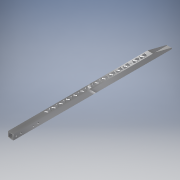
# Autodesk Inventor part: 15102898-16-P-0216
Saved by Autodesk Inventor 2017 (Build 210142000, 142)
## iProperties
Created: 2016-10-06
Part Number: 15102898-16-P-0216
Material: Aluminum 6061
Document SubType Name: Modeling
Designer: gus
Density: 2.7 g/cm^3
Appearance: Aluminum - Flat
Mass: 558.645 g
Surface Area: 1315.32 cm^2
Volume: 206.905 cm^3
Author: gus
Autodesk Inventor part; units mm, degrees
ref_plane "YZ Plane" through (0, 0, 0) normal (1, 0, 0) x (0, 1, 0)
ref_plane "XZ Plane" through (0, 0, 0) normal (0, 1, 0) x (-1, 0, 0)
ref_plane "XY Plane" through (0, 0, 0) normal (0, 0, 1) x (1, 0, 0)
sketch "Sketch1" plane through (0, 0, 0) normal (0, 0, 1) x (1, 0, 0)
  line L0 (0, 0) -> (-25.4, 0)
  line L1 (-25.4, 0) -> (-25.4, 25.4)
  line L2 (-25.4, 25.4) -> (0, 25.4)
  line L3 (0, 25.4) -> (0, 0)
  line L4 (-22.225, 22.225) -> (-22.225, 3.175)
  line L5 (-22.225, 3.175) -> (-3.175, 3.175)
  line L6 (-3.175, 3.175) -> (-3.175, 22.225)
  line L7 (-3.175, 22.225) -> (-22.225, 22.225)
  dimension "d0" = 25.4
  dimension "d1" = 25.4
  dimension "d2" = 3.175
  constraints: 16 end point, 4 parallel, 2 perpendicular, 1 horizontal, 3 other
  measures "d0" distance of L1.end L2.end
  measures "d1" distance of L0.end L1.end
  measures "d2" distance between parallel lines of L1 L4
extrude "Extrusion1" add sketch "Sketch1" along normal blind 736.6
sketch "Sketch2" plane through (-25.4, 25.4, 0) normal (0, 1, 0) x (1, 0, 0)
  circle A0 centre (12.7, -177.8) radius 3.175
  line L0 (0, 0) -> (0, -736.6) projected
  line L1 (0, 0) -> (25.4, 0) projected
  dimension "d5" = 6.35
  dimension "d6" = 12.7
  dimension "d7" = 177.8
  constraints: 1 centre point
  measures "d5" diameter of A0
  measures "d6" distance from line of L0 A0.centre
  measures "d7" distance from line of L1 A0.centre
extrude "Extrusion2" cut sketch "Sketch2" against normal blind 25.4
sketch "Sketch3" plane through (-25.4, 0, 0) normal (-1, 0, 0) x (0, 0, 1)
  circle A0 centre (723.9, 12.7) radius 3.175
  line L0 (0, 0) -> (736.6, 0) projected
  line L1 (736.6, 25.4) -> (736.6, 0) projected
  line L2 (736.6, 12.7) -> (584.2, 12.7) construction
  circle A1 centre (701.675, 12.7) radius 3.175
  circle A2 centre (644.525, 12.7) radius 3.175
  circle A3 centre (622.3, 12.7) radius 3.175
  dimension "d10" = 6.35
  dimension "d11" = 12.7
  dimension "d12" = 152.4
  dimension "d13" = 12.7
  dimension "d14" = 12.7
  dimension "d15" = 6.35
  dimension "d16" = 22.225
  dimension "d17" = 6.35
  dimension "d18" = 6.35
  dimension "d19" = 57.15
  dimension "d20" = 22.225
  constraints: 4 centre point, 3 point on line, 2 end point, 1 horizontal, 1 midpoint
  measures "d10" diameter of A0
  measures "d11" distance from line of L0 A0.centre
  measures "d12" distance of L2.start L2.end
  measures "d13" distance between parallel lines of L0 L2
  measures "d14" distance from line of L1 A0.centre
  measures "d15" diameter of A1
  measures "d16" distance of A0.centre A1.centre
  measures "d17" diameter of A2
  measures "d18" diameter of A3
  measures "d19" distance of A1.centre A2.centre
  measures "d20" distance of A3.centre A2.centre
extrude "Extrusion3" cut sketch "Sketch3" against normal blind 25.4
sketch "Sketch4" plane through (-25.4, 25.4, 0) normal (0, 1, 0) x (1, 0, 0)
  circle A0 centre (12.7, -723.9) radius 3.175
  circle A1 centre (12.7, -660.4) radius 3.175
  circle A2 centre (12.7, -596.9) radius 3.175
  line L0 (25.4, 0) -> (25.4, -736.6) projected
  line L1 (25.4, -736.6) -> (0, -736.6) projected
  circle A3 centre (12.7, -12.7) radius 3.175
  circle A4 centre (12.7, -92.075) radius 3.175
  line L2 (0, 0) -> (25.4, 0) projected
  line L3 (15.875, -581.4504) -> (6.2513, -575.8941)
  line L4 (6.2513, -570.3949) -> (15.875, -564.8386)
  line L5 (20.6375, -567.5882) -> (20.6375, -578.7007)
  line L6 (22.225, 0) -> (22.225, -736.6) projected
  line L7 (0, 0) -> (0, -736.6) projected
  line L8 (9.525, -564.8386) -> (19.1487, -559.2824)
  line L9 (19.1487, -553.7831) -> (9.525, -548.2268)
  line L10 (4.7625, -550.9765) -> (4.7625, -562.089)
  line L11 (22.225, 0) -> (3.175, 0) construction
  arc A5 (19.1487, -559.2824) -> (19.1487, -553.7831) centre (17.5612, -556.5327) ccw
  arc A6 (9.525, -548.2268) -> (4.7625, -550.9765) centre (7.9375, -550.9765) ccw
  arc A7 (4.7625, -562.089) -> (9.525, -564.8386) centre (7.9375, -562.089) ccw
  arc A8 (20.6375, -567.5882) -> (15.875, -564.8386) centre (17.4625, -567.5882) ccw
  arc A9 (15.875, -581.4504) -> (20.6375, -578.7007) centre (17.4625, -578.7007) ccw
  arc A10 (6.2513, -570.3949) -> (6.2513, -575.8941) centre (7.8388, -573.1445) ccw
  arc A11 (4.7625, -528.8404) -> (9.525, -531.59) centre (7.9375, -528.8404) ccw
  line L12 (4.7625, -517.7279) -> (4.7625, -528.8404)
  arc A12 (9.525, -514.9782) -> (4.7625, -517.7279) centre (7.9375, -517.7279) ccw
  arc A13 (6.2513, -537.1463) -> (6.2513, -542.6455) centre (7.8388, -539.8959) ccw
  arc A14 (20.6375, -534.3396) -> (15.875, -531.59) centre (17.4625, -534.3396) ccw
  line L13 (9.525, -531.59) -> (19.1487, -526.0338)
  line L14 (19.1487, -520.5345) -> (9.525, -514.9782)
  arc A15 (15.875, -548.2018) -> (20.6375, -545.4521) centre (17.4625, -545.4521) ccw
  line L15 (15.875, -548.2018) -> (6.2513, -542.6455)
  arc A16 (19.1487, -526.0338) -> (19.1487, -520.5345) centre (17.5612, -523.2841) ccw
  line L16 (20.6375, -534.3396) -> (20.6375, -545.4521)
  line L17 (6.2513, -537.1463) -> (15.875, -531.59)
  arc A17 (4.7625, -495.5918) -> (9.525, -498.3414) centre (7.9375, -495.5918) ccw
  line L18 (4.7625, -484.4793) -> (4.7625, -495.5918)
  arc A18 (9.525, -481.7296) -> (4.7625, -484.4793) centre (7.9375, -484.4793) ccw
  arc A19 (6.2513, -503.8977) -> (6.2513, -509.3969) centre (7.8388, -506.6473) ccw
  arc A20 (20.6375, -501.091) -> (15.875, -498.3414) centre (17.4625, -501.091) ccw
  line L19 (9.525, -498.3414) -> (19.1487, -492.7852)
  line L20 (19.1487, -487.2859) -> (9.525, -481.7296)
  arc A21 (15.875, -514.9532) -> (20.6375, -512.2035) centre (17.4625, -512.2035) ccw
  line L21 (15.875, -514.9532) -> (6.2513, -509.3969)
  arc A22 (19.1487, -492.7852) -> (19.1487, -487.2859) centre (17.5612, -490.0355) ccw
  line L22 (20.6375, -501.091) -> (20.6375, -512.2035)
  line L23 (6.2513, -503.8977) -> (15.875, -498.3414)
  arc A23 (4.7625, -462.3432) -> (9.525, -465.0928) centre (7.9375, -462.3432) ccw
  line L24 (4.7625, -451.2307) -> (4.7625, -462.3432)
  arc A24 (9.525, -448.481) -> (4.7625, -451.2307) centre (7.9375, -451.2307) ccw
  arc A25 (6.2513, -470.6491) -> (6.2513, -476.1483) centre (7.8388, -473.3987) ccw
  arc A26 (20.6375, -467.8424) -> (15.875, -465.0928) centre (17.4625, -467.8424) ccw
  line L25 (9.525, -465.0928) -> (19.1487, -459.5366)
  line L26 (19.1487, -454.0373) -> (9.525, -448.481)
  arc A27 (15.875, -481.7046) -> (20.6375, -478.9549) centre (17.4625, -478.9549) ccw
  line L27 (15.875, -481.7046) -> (6.2513, -476.1483)
  arc A28 (19.1487, -459.5366) -> (19.1487, -454.0373) centre (17.5612, -456.7869) ccw
  line L28 (20.6375, -467.8424) -> (20.6375, -478.9549)
  line L29 (6.2513, -470.6491) -> (15.875, -465.0928)
  arc A29 (4.7625, -429.0946) -> (9.525, -431.8442) centre (7.9375, -429.0946) ccw
  line L30 (4.7625, -417.9821) -> (4.7625, -429.0946)
  arc A30 (9.525, -415.2324) -> (4.7625, -417.9821) centre (7.9375, -417.9821) ccw
  arc A31 (6.2513, -437.4005) -> (6.2513, -442.8997) centre (7.8388, -440.1501) ccw
  arc A32 (20.6375, -434.5938) -> (15.875, -431.8442) centre (17.4625, -434.5938) ccw
  line L31 (9.525, -431.8442) -> (19.1487, -426.288)
  line L32 (19.1487, -420.7887) -> (9.525, -415.2324)
  arc A33 (15.875, -448.456) -> (20.6375, -445.7063) centre (17.4625, -445.7063) ccw
  line L33 (15.875, -448.456) -> (6.2513, -442.8997)
  arc A34 (19.1487, -426.288) -> (19.1487, -420.7887) centre (17.5612, -423.5383) ccw
  line L34 (20.6375, -434.5938) -> (20.6375, -445.7063)
  line L35 (6.2513, -437.4005) -> (15.875, -431.8442)
  arc A35 (4.7625, -395.846) -> (9.525, -398.5956) centre (7.9375, -395.846) ccw
  line L36 (4.7625, -384.7335) -> (4.7625, -395.846)
  arc A36 (9.525, -381.9838) -> (4.7625, -384.7335) centre (7.9375, -384.7335) ccw
  arc A37 (6.2513, -404.1519) -> (6.2513, -409.6511) centre (7.8388, -406.9015) ccw
  arc A38 (20.6375, -401.3452) -> (15.875, -398.5956) centre (17.4625, -401.3452) ccw
  line L37 (9.525, -398.5956) -> (19.1487, -393.0394)
  line L38 (19.1487, -387.5401) -> (9.525, -381.9838)
  arc A39 (15.875, -415.2074) -> (20.6375, -412.4577) centre (17.4625, -412.4577) ccw
  line L39 (15.875, -415.2074) -> (6.2513, -409.6511)
  arc A40 (19.1487, -393.0394) -> (19.1487, -387.5401) centre (17.5612, -390.2897) ccw
  line L40 (20.6375, -401.3452) -> (20.6375, -412.4577)
  line L41 (6.2513, -404.1519) -> (15.875, -398.5956)
  arc A41 (4.7625, -362.5974) -> (9.525, -365.347) centre (7.9375, -362.5974) ccw
  line L42 (4.7625, -351.4849) -> (4.7625, -362.5974)
  arc A42 (9.525, -348.7352) -> (4.7625, -351.4849) centre (7.9375, -351.4849) ccw
  arc A43 (6.2513, -370.9033) -> (6.2513, -376.4025) centre (7.8388, -373.6529) ccw
  arc A44 (20.6375, -368.0966) -> (15.875, -365.347) centre (17.4625, -368.0966) ccw
  line L43 (9.525, -365.347) -> (19.1487, -359.7908)
  line L44 (19.1487, -354.2915) -> (9.525, -348.7352)
  arc A45 (15.875, -381.9588) -> (20.6375, -379.2091) centre (17.4625, -379.2091) ccw
  line L45 (15.875, -381.9588) -> (6.2513, -376.4025)
  arc A46 (19.1487, -359.7908) -> (19.1487, -354.2915) centre (17.5612, -357.0411) ccw
  line L46 (20.6375, -368.0966) -> (20.6375, -379.2091)
  line L47 (6.2513, -370.9033) -> (15.875, -365.347)
  arc A47 (4.7625, -329.3488) -> (9.525, -332.0984) centre (7.9375, -329.3488) ccw
  line L48 (4.7625, -318.2363) -> (4.7625, -329.3488)
  arc A48 (9.525, -315.4866) -> (4.7625, -318.2363) centre (7.9375, -318.2363) ccw
  arc A49 (6.2513, -337.6547) -> (6.2513, -343.1539) centre (7.8388, -340.4043) ccw
  arc A50 (20.6375, -334.848) -> (15.875, -332.0984) centre (17.4625, -334.848) ccw
  line L49 (9.525, -332.0984) -> (19.1487, -326.5422)
  line L50 (19.1487, -321.0429) -> (9.525, -315.4866)
  arc A51 (15.875, -348.7102) -> (20.6375, -345.9605) centre (17.4625, -345.9605) ccw
  line L51 (15.875, -348.7102) -> (6.2513, -343.1539)
  arc A52 (19.1487, -326.5422) -> (19.1487, -321.0429) centre (17.5612, -323.7925) ccw
  line L52 (20.6375, -334.848) -> (20.6375, -345.9605)
  line L53 (6.2513, -337.6547) -> (15.875, -332.0984)
  arc A53 (4.7625, -296.1002) -> (9.525, -298.8498) centre (7.9375, -296.1002) ccw
  line L54 (4.7625, -284.9877) -> (4.7625, -296.1002)
  arc A54 (9.525, -282.238) -> (4.7625, -284.9877) centre (7.9375, -284.9877) ccw
  arc A55 (6.2513, -304.4061) -> (6.2513, -309.9053) centre (7.8388, -307.1557) ccw
  arc A56 (20.6375, -301.5994) -> (15.875, -298.8498) centre (17.4625, -301.5994) ccw
  line L55 (9.525, -298.8498) -> (19.1487, -293.2936)
  line L56 (19.1487, -287.7943) -> (9.525, -282.238)
  arc A57 (15.875, -315.4616) -> (20.6375, -312.7119) centre (17.4625, -312.7119) ccw
  line L57 (15.875, -315.4616) -> (6.2513, -309.9053)
  arc A58 (19.1487, -293.2936) -> (19.1487, -287.7943) centre (17.5612, -290.5439) ccw
  line L58 (20.6375, -301.5994) -> (20.6375, -312.7119)
  line L59 (6.2513, -304.4061) -> (15.875, -298.8498)
  arc A59 (4.7625, -262.8516) -> (9.525, -265.6012) centre (7.9375, -262.8516) ccw
  line L60 (4.7625, -251.7391) -> (4.7625, -262.8516)
  arc A60 (9.525, -248.9894) -> (4.7625, -251.7391) centre (7.9375, -251.7391) ccw
  arc A61 (6.2513, -271.1575) -> (6.2513, -276.6567) centre (7.8388, -273.9071) ccw
  arc A62 (20.6375, -268.3508) -> (15.875, -265.6012) centre (17.4625, -268.3508) ccw
  line L61 (9.525, -265.6012) -> (19.1487, -260.045)
  line L62 (19.1487, -254.5457) -> (9.525, -248.9894)
  arc A63 (15.875, -282.213) -> (20.6375, -279.4633) centre (17.4625, -279.4633) ccw
  line L63 (15.875, -282.213) -> (6.2513, -276.6567)
  arc A64 (19.1487, -260.045) -> (19.1487, -254.5457) centre (17.5612, -257.2953) ccw
  line L64 (20.6375, -268.3508) -> (20.6375, -279.4633)
  line L65 (6.2513, -271.1575) -> (15.875, -265.6012)
  arc A65 (4.7625, -229.603) -> (9.525, -232.3526) centre (7.9375, -229.603) ccw
  line L66 (4.7625, -218.4905) -> (4.7625, -229.603)
  arc A66 (9.525, -215.7408) -> (4.7625, -218.4905) centre (7.9375, -218.4905) ccw
  arc A67 (6.2513, -237.9089) -> (6.2513, -243.4081) centre (7.8388, -240.6585) ccw
  arc A68 (20.6375, -235.1022) -> (15.875, -232.3526) centre (17.4625, -235.1022) ccw
  line L67 (9.525, -232.3526) -> (19.1487, -226.7964)
  line L68 (19.1487, -221.2971) -> (9.525, -215.7408)
  arc A69 (15.875, -248.9644) -> (20.6375, -246.2147) centre (17.4625, -246.2147) ccw
  line L69 (15.875, -248.9644) -> (6.2513, -243.4081)
  arc A70 (19.1487, -226.7964) -> (19.1487, -221.2971) centre (17.5612, -224.0467) ccw
  line L70 (20.6375, -235.1022) -> (20.6375, -246.2147)
  line L71 (6.2513, -237.9089) -> (15.875, -232.3526)
  arc A71 (4.7625, -196.3544) -> (9.525, -199.104) centre (7.9375, -196.3544) ccw
  line L72 (4.7625, -185.2419) -> (4.7625, -196.3544)
  arc A72 (9.525, -182.4922) -> (4.7625, -185.2419) centre (7.9375, -185.2419) ccw
  arc A73 (6.2513, -204.6603) -> (6.2513, -210.1595) centre (7.8388, -207.4099) ccw
  arc A74 (20.6375, -201.8536) -> (15.875, -199.104) centre (17.4625, -201.8536) ccw
  line L73 (9.525, -199.104) -> (19.1487, -193.5478)
  line L74 (19.1487, -188.0485) -> (9.525, -182.4922)
  arc A75 (15.875, -215.7158) -> (20.6375, -212.9661) centre (17.4625, -212.9661) ccw
  line L75 (15.875, -215.7158) -> (6.2513, -210.1595)
  arc A76 (19.1487, -193.5478) -> (19.1487, -188.0485) centre (17.5612, -190.7981) ccw
  line L76 (20.6375, -201.8536) -> (20.6375, -212.9661)
  line L77 (6.2513, -204.6603) -> (15.875, -199.104)
  line L78 (15.875, -171.3228) -> (6.2513, -165.7665)
  line L79 (6.2513, -160.2672) -> (15.875, -154.711)
  line L80 (20.6375, -157.4606) -> (20.6375, -168.5731)
  line L81 (9.525, -154.711) -> (19.1487, -149.1547)
  line L82 (19.1487, -143.6555) -> (9.525, -138.0992)
  line L83 (4.7625, -140.8489) -> (4.7625, -151.9614)
  arc A77 (6.2513, -160.2672) -> (6.2513, -165.7665) centre (7.8388, -163.0169) ccw
  arc A78 (15.875, -171.3228) -> (20.6375, -168.5731) centre (17.4625, -168.5731) ccw
  arc A79 (20.6375, -157.4606) -> (15.875, -154.711) centre (17.4625, -157.4606) ccw
  arc A80 (19.1487, -149.1547) -> (19.1487, -143.6555) centre (17.5612, -146.4051) ccw
  arc A81 (9.525, -138.0992) -> (4.7625, -140.8489) centre (7.9375, -140.8489) ccw
  arc A82 (4.7625, -151.9614) -> (9.525, -154.711) centre (7.9375, -151.9614) ccw
  line L84 (3.175, 0) -> (3.175, -736.6) projected
  arc A83 (4.7625, -118.7128) -> (9.525, -121.4624) centre (7.9375, -118.7128) ccw
  line L85 (9.525, -121.4624) -> (19.1487, -115.9061)
  arc A84 (15.875, -138.0742) -> (20.6375, -135.3245) centre (17.4625, -135.3245) ccw
  line L86 (15.875, -138.0742) -> (6.2513, -132.5179)
  arc A85 (6.2513, -127.0186) -> (6.2513, -132.5179) centre (7.8388, -129.7683) ccw
  line L87 (20.6375, -124.212) -> (20.6375, -135.3245)
  line L88 (6.2513, -127.0186) -> (15.875, -121.4624)
  arc A86 (20.6375, -124.212) -> (15.875, -121.4624) centre (17.4625, -124.212) ccw
  arc A87 (19.1487, -115.9061) -> (19.1487, -110.4069) centre (17.5612, -113.1565) ccw
  line L89 (4.7625, -107.6003) -> (4.7625, -118.7128)
  line L90 (19.1487, -110.4069) -> (9.525, -104.8506)
  arc A88 (9.525, -104.8506) -> (4.7625, -107.6003) centre (7.9375, -107.6003) ccw
  point P0 (20.6375, -584.2)
  point P1 (1.4888, -573.1445)
  point P2 (20.6375, -562.089)
  point P3 (23.9112, -556.5327)
  point P4 (4.7625, -545.4772)
  point P5 (4.7625, -567.5882)
  point P6 (4.7625, -534.3396)
  point P7 (4.7625, -512.2286)
  point P8 (23.9112, -523.2841)
  point P9 (20.6375, -550.9514)
  point P10 (1.4888, -539.8959)
  point P11 (20.6375, -528.8404)
  point P12 (4.7625, -501.091)
  point P13 (4.7625, -478.98)
  point P14 (23.9112, -490.0355)
  point P15 (20.6375, -517.7028)
  point P16 (1.4888, -506.6473)
  point P17 (20.6375, -495.5918)
  point P18 (4.7625, -467.8424)
  point P19 (4.7625, -445.7314)
  point P20 (23.9112, -456.7869)
  point P21 (20.6375, -484.4542)
  point P22 (1.4888, -473.3987)
  point P23 (20.6375, -462.3432)
  point P24 (4.7625, -434.5938)
  point P25 (4.7625, -412.4828)
  point P26 (23.9112, -423.5383)
  point P27 (20.6375, -451.2056)
  point P28 (1.4888, -440.1501)
  point P29 (20.6375, -429.0946)
  point P30 (4.7625, -401.3452)
  point P31 (4.7625, -379.2342)
  point P32 (23.9112, -390.2897)
  point P33 (20.6375, -417.957)
  point P34 (1.4888, -406.9015)
  point P35 (20.6375, -395.846)
  point P36 (4.7625, -368.0966)
  point P37 (4.7625, -345.9856)
  point P38 (23.9112, -357.0411)
  point P39 (20.6375, -384.7084)
  point P40 (1.4888, -373.6529)
  point P41 (20.6375, -362.5974)
  point P42 (4.7625, -334.848)
  point P43 (4.7625, -312.737)
  point P44 (23.9112, -323.7925)
  point P45 (20.6375, -351.4598)
  point P46 (1.4888, -340.4043)
  point P47 (20.6375, -329.3488)
  point P48 (4.7625, -301.5994)
  point P49 (4.7625, -279.4884)
  point P50 (23.9112, -290.5439)
  point P51 (20.6375, -318.2112)
  point P52 (1.4888, -307.1557)
  point P53 (20.6375, -296.1002)
  point P54 (4.7625, -268.3508)
  point P55 (4.7625, -246.2398)
  point P56 (23.9112, -257.2953)
  point P57 (20.6375, -284.9626)
  point P58 (1.4888, -273.9071)
  point P59 (20.6375, -262.8516)
  point P60 (4.7625, -235.1022)
  point P61 (4.7625, -212.9912)
  point P62 (23.9112, -224.0467)
  point P63 (20.6375, -251.714)
  point P64 (1.4888, -240.6585)
  point P65 (20.6375, -229.603)
  point P66 (4.7625, -201.8536)
  point P67 (4.7625, -179.7426)
  point P68 (23.9112, -190.7981)
  point P69 (20.6375, -218.4654)
  point P70 (1.4888, -207.4099)
  point P71 (20.6375, -196.3544)
  dimension "d23" = 63.5
  dimension "d24" = 63.5
  dimension "d25" = 6.35
  dimension "d26" = 12.7
  dimension "d27" = 12.7
  dimension "d28" = 12.7
  dimension "d29" = 12.7
  dimension "d32" = 6.35
  dimension "d33" = 6.35
  dimension "d34" = 12.7
  dimension "d35" = 92.075
  dimension "d36" = 12.7
  dimension "d37" = 12.7
  dimension "d40" = 152.4
  dimension "d58" = 3.175
  dimension "d59" = 3.175
  dimension "d60" = 11.1125
  dimension "d62" = 4.7625
  dimension "d63" = 1.5875
  dimension "d66" = 33.2486
  dimension "d73" = 3.175
  dimension "d74" = 11.1125
  dimension "d75" = 3.175
  dimension "d76" = 1.5875
  dimension "d77" = 1.5875
  dimension "d78" = 22.225
  dimension "d81" = 33.2486
  constraints: 168 end point, 168 point on circle, 156 point on line, 89 centre point, 24 tangent, 12 equal radius, 10 equal length, 4 vertical, 2 parallel, 426 other
  measures "d23" distance of A1.centre A2.centre
  measures "d24" distance of A0.centre A1.centre
  measures "d25" diameter of A2
  measures "d26" distance from line of L0 A2.centre
  measures "d27" distance from line of L0 A1.centre
  measures "d28" distance from line of L0 A0.centre
  measures "d29" distance from line of L1 A0.centre
  measures "d32" diameter of A3
  measures "d33" diameter of A4
  measures "d34" distance from line of L2 A3.centre
  measures "d35" distance from line of L2 A4.centre
  measures "d36" distance from line of L0 A4.centre
  measures "d37" distance from line of L0 A3.centre
  measures "d40" distance from line of L1 point (20.637, -584.2)
  measures "d58" radius of A5
  measures "d59" distance between parallel lines of L8 L4
  measures "d60" distance of A10.centre A8.centre
  measures "d62" distance between parallel lines of L7 L10
  measures "d63" distance between parallel lines of L6 L5
  measures "d66" distance of A8.centre A14.centre
  measures "d73" radius of A77
  measures "d74" distance of A82.centre A80.centre
  measures "d75" distance between parallel lines of L81 L79
  measures "d76" distance between parallel lines of L84 L83
  measures "d77" distance between parallel lines of L6 L80
  measures "d78" vertical distance of A76.centre A78.centre
  measures "d81" distance of L78.end L86.end
extrude "Extrusion6" cut sketch "Sketch4" against normal blind 25.4 contours A3 | A4 | L3 A10 L4 A8 L5 A9 | A7 L10 A6 L9 A5 L8 | L12 A12 L14 A16 L13 A11 | L17 A14 L16 A15 L15 A13 | L18 A18 L20 A22 L19 A17 | L23 A20 L22 A21 L21 A19 | L24 A24 L26 A28 L25 A23 | L29 A26 L28 A27 L27 A25 | L30 A30 L32 A34 L31 A29 | L35 A32 L34 A33 L33 A31 | L36 A36 L38 A40 L37 A35 | L41 A38 L40 A39 L39 A37 | L42 A42 L44 A46 L43 A41 | L47 A44 L46 A45 L45 A43 | L48 A48 L50 A52 L49 A47 | L53 A50 L52 A51 L51 A49 | L54 A54 L56 A58 L55 A53 | L59 A56 L58 A57 L57 A55 | L60 A60 L62 A64 L61 A59 | L65 A62 L64 A63 L63 A61 | L66 A66 L68 A70 L67 A65 | L71 A68 L70 A69 L69 A67 | L72 A72 L74 A76 L73 A71 | L77 A74 L76 A75 L75 A73 | L78 A77 L79 A79 L80 A78 | A82 L83 A81 L82 A80 L81 | L89 A88 L90 A87 L85 A83 | L86 A85 L88 A86 L87 A84
sketch "Sketch5" plane through (-25.4, 0, 0) normal (-1, 0, 0) x (0, 0, 1)
  line L0 (0, 0) -> (0, 25.4) projected
  line L1 (0, 3.175) -> (88.9, 25.4)
  line L2 (88.9, 25.4) -> (0, 25.4)
  line L3 (0, 0) -> (736.6, 0) projected
  dimension "d86" = 22.225
  dimension "d87" = 88.9
  constraints: 4 end point, 1 parallel, 1 point on line
  measures "d86" distance of L0.end L1.start
  measures "d87" distance of L1.end L0.end
extrude "Extrusion7" cut sketch "Sketch5" against normal blind 25.4
body "Solid1"
